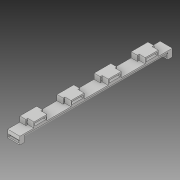
# Autodesk Inventor part: Rystyset 1,0 v2
Saved by Autodesk Inventor 2019 (Build 230136000, 136)
## iProperties
Created: 2018-07-23
Part Number: Rystyset 1,0 v2
Material: Generic
Document SubType Name: Modeling
Designer: sakki
Density: 1 g/cm^3
Appearance: Default
Author: sakki
## iProperties of the stored document Rystyset 1,0 v2_3DPrint.ipt
Created: 2018-07-23
Part Number: Rystyset 1,0 v2_3DPrint
Material: Generic
Document SubType Name: Modeling
Designer: sakki
Density: 1 g/cm^3
Appearance: Default
Author: sakki
Autodesk Inventor part; units mm, degrees
ref_plane "YZ Plane" through (0, 0, 0) normal (1, 0, 0) x (0, 1, 0)
ref_plane "XZ Plane" through (0, 0, 0) normal (0, 1, 0) x (-1, 0, 0)
ref_plane "XY Plane" through (0, 0, 0) normal (0, 0, 1) x (1, 0, 0)
sketch "Sketch1" plane through (0, 0, 0) normal (0, 1, 0) x (-1, 0, 0)
  line L0 (0, 0) -> (-8, 0)
  line L1 (-8, 0) -> (-8, 120)
  line L2 (-8, 120) -> (0, 120)
  line L3 (0, 120) -> (0, 0)
  dimension "d0" = 8
  dimension "d1" = 120
  constraints: 8 end point, 2 parallel, 1 horizontal, 1 perpendicular
  measures "d0" distance of L1.end L2.end
  measures "d1" distance of L0.end L1.end
extrude "Extrusion1" add sketch "Sketch1" along normal blind 2.5
sketch "Sketch2" plane through (0, 2.5, 0) normal (0, 1, 0) x (1, 0, 0)
  line L0 (0, 0) -> (0, -120) projected
  line L1 (0, -120) -> (0, -112)
  line L2 (0, 0) -> (0, -28)
  line L3 (0, -112) -> (0, -101)
  line L4 (0, -101) -> (0, -87.667)
  line L5 (0, -87.667) -> (0, -76.667)
  line L6 (0, -76.667) -> (0, -63.334)
  line L7 (0, -63.334) -> (0, -52.334)
  line L8 (0, -52.334) -> (0, -39.001)
  line L9 (0, -39.001) -> (0, -28)
  line L10 (0, -120) -> (8, -120) projected
  line L11 (8, -120) -> (8, -110.778)
  line L12 (8, -120) -> (8, 0) projected
  line L13 (8, -110.778) -> (8, -102.222)
  line L14 (8, -102.222) -> (8, -86.445)
  line L15 (8, -86.445) -> (8, -77.889)
  line L16 (8, -77.889) -> (8, -62.112)
  line L17 (8, -62.112) -> (8, -53.556)
  line L18 (8, -53.556) -> (8, -37.779)
  line L19 (8, -37.779) -> (8, -29.223)
  line L20 (8, -29.223) -> (8, 0)
  line L21 (0, -120) -> (4, -120)
  line L22 (0, 0) -> (4, 0)
  line L23 (8, 0) -> (0, 0) projected
  line L24 (4, 0) -> (4, -120)
  line L25 (0, -101) -> (4, -101)
  line L26 (0, -112) -> (4, -112)
  line L27 (4, -112) -> (4, -110.778)
  line L28 (8, -110.778) -> (4, -110.778)
  line L29 (4, -101) -> (4, -102.222)
  line L30 (8, -102.222) -> (4, -102.222)
  line L31 (8, -102.222) -> (8, -110.778)
  line L32 (0, -112) -> (0, -101)
  line L33 (4, -112) -> (4, -110.778)
  line L34 (0, -87.667) -> (0, -76.667)
  line L35 (4, -76.667) -> (0, -76.667)
  line L36 (4, -76.667) -> (4, -77.889)
  line L37 (8, -77.889) -> (4, -77.889)
  line L38 (8, -77.889) -> (8, -86.445)
  line L39 (8, -86.445) -> (4, -86.445)
  line L40 (4, -86.445) -> (4, -87.667)
  line L41 (4, -87.667) -> (0, -87.667)
  line L42 (0, -63.334) -> (4, -63.334)
  line L43 (4, -63.334) -> (4, -62.112)
  line L44 (4, -62.112) -> (8, -62.112)
  line L45 (8, -62.112) -> (8, -53.556)
  line L46 (8, -53.556) -> (4, -53.556)
  line L47 (4, -53.556) -> (4, -52.334)
  line L48 (4, -52.334) -> (0, -52.334)
  line L49 (0, -52.334) -> (0, -63.334)
  line L50 (0, -39.001) -> (4, -39.001)
  line L51 (4, -39.001) -> (4, -37.779)
  line L52 (4, -37.779) -> (8, -37.779)
  line L53 (8, -37.779) -> (8, -29.223)
  line L54 (8, -29.223) -> (4, -29.223)
  line L55 (4, -29.223) -> (4, -28)
  line L56 (4, -28) -> (0, -28)
  line L57 (0, -28) -> (0, -39.001)
  dimension "d4" = 8
  dimension "d5" = 28
  dimension "d6" = 11
  dimension "d7" = 13.333
  dimension "d8" = 11
  dimension "d9" = 13.333
  dimension "d10" = 11
  dimension "d11" = 13.333
  dimension "d12" = 11.001
  dimension "d13" = 9.222
  dimension "d14" = 8.556
  dimension "d15" = 15.777
  dimension "d16" = 8.556
  dimension "d17" = 15.777
  dimension "d18" = 8.556
  dimension "d19" = 15.777
  dimension "d20" = 8.556
  dimension "d21" = 29.223
  dimension "d93" = 1.223
  constraints: 106 end point, 14 perpendicular, 6 horizontal, 5 vertical, 2 midpoint, 2 parallel, 1 collinear, 37 other
  measures "d4" distance of L1.start L1.end
  measures "d5" distance of L2.start L2.end
  measures "d6" distance of L1.end L3.end
  measures "d7" distance of L3.end L4.end
  measures "d8" distance of L4.end L5.end
  measures "d9" distance of L5.end L6.end
  measures "d10" distance of L6.end L7.end
  measures "d11" distance of L7.end L8.end
  measures "d12" distance of L8.end L2.end
  measures "d13" distance of L10.end L11.end
  measures "d14" distance of L11.end L13.end
  measures "d15" distance of L13.end L14.end
  measures "d16" distance of L14.end L15.end
  measures "d17" distance of L15.end L16.end
  measures "d18" distance of L16.end L17.end
  measures "d19" distance of L17.end L18.end
  measures "d20" distance of L18.end L19.end
  measures "d21" distance of L19.end L20.end
  measures "d93" distance of L54.end L55.end
extrude "Extrusion2" add sketch "Sketch2" along normal blind 3.5 contours L56 L24 L50 L0 | L48 L24 L42 L0 | L54 L12 L52 L24 | L35 L24 L41 L0 | L46 L12 L44 L24 | L25 L24 L26 L0 | L37 L12 L39 L24 | L30 L12 L28 L24
sketch "Sketch3" plane through (8, 0, 120) normal (1, 0, 0) x (0, 0, -1)
  line L0 (90.777, 2.5) -> (90.777, 6) projected
  line L1 (90.777, 2.5) -> (90.777, 3.4)
  line L2 (90.777, 3.4) -> (90.149, 3.4)
  line L3 (82.221, 2.5) -> (82.221, 6) projected
  line L4 (82.221, 6) -> (82.221, 5.1)
  line L5 (82.221, 5.1) -> (82.849, 5.1)
  line L6 (82.849, 5.1) -> (90.149, 5.1)
  line L7 (90.149, 5.1) -> (90.149, 3.4)
  line L8 (90.149, 3.4) -> (82.849, 3.4)
  line L9 (82.849, 3.4) -> (82.849, 5.1)
  point P0 (120, 0)
  dimension "d25" = 0.9
  dimension "d26" = 0.628
  dimension "d27" = 0.9
  dimension "d28" = 0.628
  constraints: 16 end point, 3 horizontal, 2 parallel, 2 point on line, 1 perpendicular
  measures "d25" distance of L0.start L1.end
  measures "d26" distance of L1.end L2.end
  measures "d27" distance of L3.end L4.end
  measures "d28" distance of L4.end L5.end
extrude "Extrusion3" cut sketch "Sketch3" against normal blind 4
sketch "Sketch4" plane through (0, 0, 0) normal (-1, 0, 0) x (0, 0, 1)
  line L0 (28, 2.5) -> (28, 6) projected
  line L1 (28, 6) -> (28, 5.1)
  line L2 (39.001, 2.5) -> (39.001, 6) projected
  line L3 (39.001, 2.5) -> (39.001, 3.4)
  line L4 (39.001, 3.4) -> (38.373, 3.4)
  line L5 (37.779, 2.5) -> (37.779, 6) projected
  line L6 (28, 5.1) -> (28.628, 5.1)
  line L7 (28.628, 5.1) -> (38.373, 5.1)
  line L8 (38.373, 5.1) -> (38.373, 3.4)
  line L9 (38.373, 3.4) -> (28.628, 3.4)
  line L10 (28.628, 3.4) -> (28.628, 5.1)
  point P0 (0, 0)
  dimension "d31" = 0.9
  dimension "d32" = 0.9
  dimension "d33" = 0.628
  dimension "d34" = 0.628
  constraints: 16 end point, 2 horizontal, 2 parallel, 2 perpendicular, 2 point on line
  measures "d31" distance of L0.end L1.end
  measures "d32" distance of L2.start L3.end
  measures "d33" distance of L3.end L4.end
  measures "d34" distance of L1.end L6.end
extrude "Extrusion4" cut sketch "Sketch4" against normal blind 4
sketch "Sketch6" plane through (0, 0, 0) normal (0, -1, 0) x (1, 0, 0)
  line L0 (0, 0) -> (8, 0) projected
  line L1 (8, 0) -> (0, 0)
  line L2 (0, 0) -> (0, 3)
  line L3 (0, 3) -> (8, 3)
  line L4 (8, 3) -> (8, 0)
  line L5 (8, 120.0098) -> (0, 120.0098)
  line L6 (0, 120.0098) -> (0, 117.0098)
  line L7 (0, 117.0098) -> (8, 117.0098)
  line L8 (8, 117.0098) -> (8, 120.0098)
  dimension "d37" = 8
  dimension "d38" = 3
  dimension "d39" = 8
  dimension "d40" = 3
  constraints: 16 end point, 4 parallel, 2 horizontal, 2 perpendicular
  measures "d37" distance of L2.end L3.end
  measures "d38" distance of L1.end L2.end
  measures "d39" distance of L7.end L6.end
  measures "d40" distance of L6.end L5.end
extrude "Extrusion5" add sketch "Sketch6" along normal blind 2.5
sketch "Sketch7" plane through (8, 2.5, 0) normal (0, 0, -1) x (-1, 0, 0)
  line L0 (8, -5) -> (8, 0) projected
  line L1 (8, -5) -> (8, -4.1)
  line L2 (8, -4.1) -> (7.372, -4.1)
  line L3 (7.372, -4.1) -> (0.628, -4.1)
  line L4 (0.628, -4.1) -> (0.628, -2.738)
  line L5 (0.628, -2.738) -> (7.372, -2.738)
  line L6 (7.372, -2.738) -> (7.372, -4.1)
  point P0 (8, -2.5)
  dimension "d43" = 0.9
  dimension "d44" = 0.628
  dimension "d45" = 6.744
  dimension "d46" = 1.362
  constraints: 12 end point, 2 parallel, 2 perpendicular, 1 horizontal, 1 point on line
  measures "d43" distance of L0.start L1.end
  measures "d44" distance of L1.end L2.end
  measures "d45" distance of L4.end L5.end
  measures "d46" distance of L3.end L4.end
extrude "Extrusion6" cut sketch "Sketch7" against normal blind 3
sketch "Sketch8" plane through (0, 0, 120.0098) normal (0, 0, 1) x (1, 0, 0)
  line L0 (8, 2.5) -> (8, -2.5) projected
  line L1 (8, -2.5) -> (8, -1.6)
  line L2 (8, -1.6) -> (7.372, -1.6)
  line L3 (7.372, -1.6) -> (0.628, -1.6) projected
  line L4 (0.628, -0.238) -> (7.372, -0.238) projected
  line L5 (7.372, -1.6) -> (0.628, -1.6)
  line L6 (0.628, -1.6) -> (0.628, -0.238)
  line L7 (0.628, -0.238) -> (7.372, -0.238)
  line L8 (7.372, -0.238) -> (7.372, -1.6)
  point P0 (0, 0)
  dimension "d49" = 0.9
  dimension "d50" = 0.628
  constraints: 12 end point, 2 parallel, 2 perpendicular, 1 horizontal, 1 point on line
  measures "d49" distance of L0.end L1.end
  measures "d50" distance of L1.end L2.end
extrude "Extrusion7" cut sketch "Sketch8" against normal blind 3
sketch "Sketch9" plane through (0, 2.5, 112) normal (-1, 0, 0) x (0, 0, 1)
  line L0 (-59.666, 3.5) -> (-48.666, 3.5) projected
  line L1 (-59.666, 3.5) -> (-59.666, 2.6)
  line L2 (-59.666, 0) -> (-59.666, 3.5) projected
  line L3 (-59.666, 2.6) -> (-59.038, 2.6)
  line L4 (-48.666, 0) -> (-48.666, 3.5) projected
  line L5 (-48.666, 0) -> (-48.666, 0.9)
  line L6 (-48.666, 0.9) -> (-49.294, 0.9)
  line L7 (-59.038, 2.6) -> (-49.294, 2.6)
  line L8 (-49.294, 2.6) -> (-49.294, 0.9)
  line L9 (-49.294, 0.9) -> (-59.038, 0.9)
  line L10 (-59.038, 0.9) -> (-59.038, 2.6)
  point P0 (-112, -2.5)
  dimension "d53" = 0.9
  dimension "d54" = 0.628
  dimension "d55" = 0.9
  dimension "d56" = 0.628
  constraints: 16 end point, 3 perpendicular, 2 parallel, 2 point on line, 1 horizontal
  measures "d53" distance of L0.start L1.end
  measures "d54" distance of L1.end L3.end
  measures "d55" distance of L4.start L5.end
  measures "d56" distance of L5.end L6.end
extrude "Extrusion8" cut sketch "Sketch9" against normal blind 4 contours L7 L8 L9 L10
sketch "Sketch10" plane through (8, 2.5, 29.223) normal (1, 0, 0) x (0, 0, -1)
  line L0 (-32.889, 3.5) -> (-32.889, 2.6)
  line L1 (-32.889, 0) -> (-32.889, 3.5) projected
  line L2 (-32.889, 2.6) -> (-32.261, 2.6)
  line L3 (-23.739, 2.6) -> (-33.483, 2.6) projected
  line L4 (-24.333, 0) -> (-24.333, 3.5) projected
  line L5 (-24.333, 0) -> (-24.333, 0.9)
  line L6 (-24.333, 0.9) -> (-24.961, 0.9)
  line L7 (-32.889, 0.9) -> (-24.333, 0.9) projected
  line L8 (-32.261, 2.6) -> (-24.961, 2.6)
  line L9 (-24.961, 2.6) -> (-24.961, 0.9)
  line L10 (-24.961, 0.9) -> (-32.261, 0.9)
  line L11 (-32.261, 0.9) -> (-32.261, 2.6)
  point P0 (29.223, -2.5)
  dimension "d59" = 0.9
  dimension "d60" = 0.628
  dimension "d62" = 0.628
  constraints: 16 end point, 4 point on line, 2 parallel, 1 horizontal, 1 perpendicular
  measures "d59" distance of L0.start L0.end
  measures "d60" distance of L0.end L2.end
  measures "d62" distance of L5.end L6.end
extrude "Extrusion9" cut sketch "Sketch10" against normal blind 4 contours L11 L3 L9 L7
sketch "Sketch11" plane through (8, 2.5, 29.223) normal (1, 0, 0) x (0, 0, -1)
  line L0 (-57.222, 0) -> (-57.222, 3.5) projected
  line L1 (-57.222, 3.5) -> (-57.222, 2.6)
  line L2 (-57.222, 2.6) -> (-56.594, 2.6)
  line L3 (-48.666, 0) -> (-32.889, 0) projected
  line L4 (-48.666, 0) -> (-48.666, 0.9)
  line L5 (-48.666, 0) -> (-48.666, 3.5) projected
  line L6 (-48.666, 0.9) -> (-48.666, 0.272)
  line L7 (-56.594, 2.6) -> (-49.294, 2.6)
  line L8 (-49.294, 2.6) -> (-49.294, 0.9)
  line L9 (-49.294, 0.9) -> (-56.594, 0.9)
  line L10 (-56.594, 0.9) -> (-56.594, 2.6)
  point P0 (29.223, -2.5)
  dimension "d65" = 0.9
  dimension "d66" = 0.628
  dimension "d67" = 0.9
  dimension "d68" = 0.628
  dimension "d69" = 7.3
  constraints: 16 end point, 3 point on line, 2 parallel, 2 perpendicular, 1 horizontal
  measures "d65" distance of L0.end L1.end
  measures "d66" distance of L1.end L2.end
  measures "d67" distance of L3.start L4.end
  measures "d68" distance of L4.end L6.end
  measures "d69" distance of L8.end L9.end
extrude "Extrusion10" cut sketch "Sketch11" against normal blind 4
sketch "Sketch12" plane through (0, 2.5, 112) normal (-1, 0, 0) x (0, 0, 1)
  line L0 (-35.333, 0) -> (-35.333, 3.5) projected
  line L1 (-35.333, 3.5) -> (-35.333, 2.6)
  line L2 (-35.333, 2.6) -> (-34.705, 2.6)
  line L3 (-24.333, 0) -> (-24.333, 3.5) projected
  line L4 (-24.333, 0) -> (-24.333, 0.9)
  line L5 (-24.333, 0.9) -> (-24.333, 0.272)
  line L6 (-24.333, 0.9) -> (-24.961, 0.9)
  line L7 (-34.705, 2.6) -> (-24.961, 2.6)
  line L8 (-24.961, 2.6) -> (-24.961, 0.9)
  line L9 (-24.961, 0.9) -> (-34.705, 0.9)
  line L10 (-34.705, 0.9) -> (-34.705, 2.6)
  point P0 (-112, -2.5)
  dimension "d72" = 0.9
  dimension "d73" = 0.628
  dimension "d74" = 0.9
  dimension "d75" = 0.628
  dimension "d76" = 0.628
  constraints: 18 end point, 3 point on line, 2 horizontal, 2 parallel, 2 perpendicular
  measures "d72" distance of L0.end L1.end
  measures "d73" distance of L1.end L2.end
  measures "d74" distance of L3.start L4.end
  measures "d75" distance of L4.end L5.end
  measures "d76" distance of L4.end L6.end
extrude "Extrusion11" cut sketch "Sketch12" against normal blind 4
sketch "Sketch13" plane through (0, 2.5, 112) normal (-1, 0, 0) x (0, 0, 1)
  line L0 (-11, 3.5) -> (-11, 2.6)
  line L1 (-11, 0) -> (-11, 3.5) projected
  line L2 (-11, 2.6) -> (-10.372, 2.6)
  line L3 (0, 0) -> (8, 0) projected
  line L4 (0, 0) -> (0, 0.9)
  line L5 (0, 0.9) -> (-0.628, 0.9)
  line L6 (-10.372, 2.6) -> (-0.628, 2.6)
  line L7 (-0.628, 2.6) -> (-0.628, 0.9)
  line L8 (-0.628, 0.9) -> (-10.372, 0.9)
  line L9 (-10.372, 0.9) -> (-10.372, 2.6)
  point P0 (-112, -2.5)
  dimension "d79" = 0.9
  dimension "d80" = 0.628
  dimension "d81" = 0.9
  dimension "d82" = 0.628
  constraints: 16 end point, 3 perpendicular, 2 horizontal, 2 parallel, 1 point on line
  measures "d79" distance of L0.start L0.end
  measures "d80" distance of L0.end L2.end
  measures "d81" distance of L3.start L4.end
  measures "d82" distance of L4.end L5.end
extrude "Extrusion12" cut sketch "Sketch13" against normal blind 4
sketch "Sketch14" plane through (8, 2.5, 29.223) normal (1, 0, 0) x (0, 0, -1)
  line L0 (-81.555, 0) -> (-81.555, 3.5) projected
  line L1 (-81.555, 3.5) -> (-81.555, 2.6)
  line L2 (-81.555, 2.6) -> (-80.927, 2.6)
  line L3 (-72.999, 2.6) -> (-81.555, 2.6) projected
  line L4 (-72.999, 0) -> (-72.999, 3.5) projected
  line L5 (-72.999, 0) -> (-72.999, 0.9)
  line L6 (-72.999, 0.9) -> (-73.627, 0.9)
  line L7 (-81.555, 0.9) -> (-72.999, 0.9) projected
  line L8 (-80.927, 2.6) -> (-73.627, 2.6)
  line L9 (-73.627, 2.6) -> (-73.627, 0.9)
  line L10 (-73.627, 0.9) -> (-80.927, 0.9)
  line L11 (-80.927, 0.9) -> (-80.927, 2.6)
  point P0 (29.223, -2.5)
  dimension "d86" = 0.628
  dimension "d88" = 0.628
  constraints: 16 end point, 4 point on line, 2 parallel, 1 horizontal, 1 perpendicular
  measures "d86" distance of L1.end L2.end
  measures "d88" distance of L5.end L6.end
extrude "Extrusion13" cut sketch "Sketch14" against normal blind 4 contours L11 L3 L9 L7
sketch "Sketch15" plane through (0, 2.5, 0) normal (0, 1, 0) x (1, 0, 0)
  line L0 (0, -28) -> (4, -28) projected
  line L1 (0, -28) -> (0, -20)
  line L2 (0, -117.0098) -> (0, -3) projected
  line L3 (0, -20) -> (8, -20)
  line L4 (8, -3) -> (8, -117.0098) projected
  line L5 (0, -20) -> (8, -20)
  line L6 (8, -20) -> (8, 0)
  line L7 (8, 0) -> (0, 0)
  line L8 (0, 0) -> (0, -20)
  dimension "d94" = 8
  constraints: 12 end point, 2 horizontal, 2 parallel, 2 point on line, 1 perpendicular
  measures "d94" distance of L0.start L1.end
extrude "Extrusion14" cut sketch "Sketch15" against normal blind 10
sketch "Sketch16" plane through (0, 0, 0) normal (0, -1, 0) x (1, 0, 0)
  line L0 (8, 20) -> (8, 117.0098) projected
  line L1 (8, 20) -> (0, 20)
  line L2 (0, 20) -> (0, 23)
  line L3 (0, 23) -> (8, 23)
  line L4 (8, 23) -> (8, 20)
  point P0 (0, 0)
  dimension "d97" = 8
  dimension "d98" = 3
  constraints: 8 end point, 2 parallel, 1 horizontal, 1 perpendicular
  measures "d97" distance of L2.end L3.end
  measures "d98" distance of L1.end L2.end
extrude "Extrusion15" add sketch "Sketch16" along normal blind 2.5
sketch "Sketch17" plane through (8, 2.5, 20) normal (0, 0, -1) x (-1, 0, 0)
  line L0 (0, -2.5) -> (0, -5) projected
  line L1 (0, -5) -> (0, -4.1)
  line L2 (0.628, -4.1) -> (7.372, -4.1) projected
  line L3 (0, -4.1) -> (0.628, -4.1)
  line L4 (0.628, -4.1) -> (0.628, -2.738) projected
  line L5 (0, -2.5) -> (8, -2.5) projected
  line L6 (0.628, -4.1) -> (7.372, -4.1)
  line L7 (7.372, -4.1) -> (7.372, -2.5)
  line L8 (7.372, -2.5) -> (0.628, -2.5)
  line L9 (0.628, -2.5) -> (0.628, -4.1)
  dimension "d101" = 0.9
  dimension "d102" = 0.628
  constraints: 12 end point, 2 parallel, 2 point on line, 1 horizontal, 1 perpendicular
  measures "d101" distance of L0.end L1.end
  measures "d102" distance of L1.end L2.start
extrude "Extrusion16" cut sketch "Sketch17" against normal blind 3 contours L5 L7 L2 L4 L9
fillet "Fillet3" radius 1.5 1 edges at (8, 0, 70.0049)
fillet "Fillet4" radius 1.5 1 edges at (0, 0, 70.0049)
body "Solid1"
